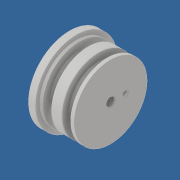
# Autodesk Inventor part: Innenflansch
Saved by Autodesk Inventor 2018 (Build 220112000, 112)
## iProperties
Created: 2018-10-02
Part Number: Innenflansch
Material: Generisch
Document SubType Name: Modeling
Designer: M.Knabel
Density: 1 g/cm^3
Appearance: Vorgabe
Author: M.Knabel
Autodesk Inventor part; units mm, degrees
ref_plane "YZ Plane" through (0, 0, 0) normal (1, 0, 0) x (0, 1, 0)
ref_plane "XZ Plane" through (0, 0, 0) normal (0, 1, 0) x (-1, 0, 0)
ref_plane "XY Plane" through (0, 0, 0) normal (0, 0, 1) x (1, 0, 0)
sketch "Skizze1" plane through (0, 0, 0) normal (0, 0, 1) x (1, 0, 0)
  line L0 (-2.4, 0) -> (14.4, 0) projected
  line L1 (0, -2.4) -> (0, 14.4) projected
  line L2 (0, 5) -> (7, 5)
  line L3 (7, 5) -> (7, 0)
  line L4 (7, 0) -> (12, 0)
  line L5 (12, 0) -> (12, 10.7)
  line L6 (12, 10.7) -> (11, 10.7)
  line L7 (11, 10.7) -> (11, 8.5)
  line L8 (11, 8.5) -> (8.5, 8.5)
  line L9 (8.5, 8.5) -> (8.5, 10.7)
  line L10 (8.5, 10.7) -> (5.4, 10.7)
  line L11 (5.4, 10.7) -> (5.4, 8.5)
  line L12 (5.4, 8.5) -> (2.9, 8.5)
  line L13 (2.9, 8.5) -> (2.9, 10.7)
  line L14 (2.9, 10.7) -> (2, 10.7)
  line L15 (2, 10.7) -> (2, 12)
  line L16 (2, 12) -> (0, 12)
  line L17 (0, 12) -> (0, 5)
  point P0 (0, 0)
  dimension "d0" = 24
  dimension "d1" = 10
  dimension "d2" = 17
  dimension "d3" = 21.4
  dimension "d4" = 2.5
  dimension "d5" = 2.5
  dimension "d7" = 1
  dimension "d8" = 6.6
  dimension "d9" = 12
  dimension "d11" = 10
  dimension "d12" = 7
  constraints: 32 end point, 10 perpendicular, 10 point on line, 1 collinear, 1 vertical
  measures "d0" diameter of L16 L0
  measures "d1" diameter of L2 L0
  measures "d2" diameter of L12 L0
  measures "d3" diameter of L10 L0
  measures "d4" distance between parallel lines of L11 L13
  measures "d5" distance between parallel lines of L7 L9
  measures "d7" distance between parallel lines of L5 L7
  measures "d8" distance between parallel lines of L5 L11
  measures "d9" distance between parallel lines of L5 L1
  measures "d11" distance between parallel lines of L15 L5
  measures "d12" distance between parallel lines of L3 L1
revolve "Umdrehung1" add sketch "Skizze1" angle 360 about axis through (-10, 0, 0) along (1, 0, 0) contours L3 L2 L1 L16 L15 L14 L13 L12 L11 L10 L9 L8 L7 L6 L5 L0
sketch "Skizze2" plane through (7, 0, 0) normal (-1, 0, 0) x (0, 0, 1)
  point P0 (0, 0)
  point P1 (0, 0)
  constraints: 1 coincident
hole "Bohrung1" at (7, 0, 0) direction (1, 0, 0) diameter 2.459 end through all countersink diameter 3.5 countersink angle 90 thread size "M3x0.5" class "6H" standard "ISO Metric profile"
sketch "Skizze3" plane through (7, 0, 0) normal (-1, 0, 0) x (0, 0, 1)
  line L0 (-16.8, 0) -> (16.8, 0) projected
  line L1 (0, -16.8) -> (0, 16.8) projected
  circle A0 centre (0, 0) radius 5 projected
  point P0 (0, 4.25)
  dimension "d21" = 4.25
  constraints: 1 point on line
  measures "d21" distance of point (0, 4.25) A0.centre
hole "Bohrung2" at (7, 4.25, 0) direction (1, 0, 0) diameter 1.5 end through all
